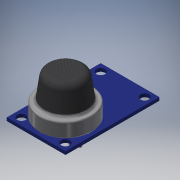
# Autodesk Inventor part: MQ_New
Saved by Autodesk Inventor 2019 (Build 230136000, 136)
## iProperties
Created: 2019-06-20
Part Number: MQ_New
Material: Steel, Mild, Welded
Document SubType Name: Modeling
Designer: hecto
Density: 7.85 g/cm^3
Appearance: Rubber - Blue(2)
Author: hecto
Autodesk Inventor part; units mm, degrees
ref_plane "YZ Plane" through (0, 0, 0) normal (1, 0, 0) x (0, 1, 0)
ref_plane "XZ Plane" through (0, 0, 0) normal (0, 1, 0) x (-1, 0, 0)
ref_plane "XY Plane" through (0, 0, 0) normal (0, 0, 1) x (1, 0, 0)
sketch "Sketch1" plane through (0, 0, 0) normal (0, 1, 0) x (-1, 0, 0)
  line L0 (10, -16) -> (-10, -16)
  line L1 (-10, -16) -> (-10, 16)
  line L2 (-10, 16) -> (10, 16)
  line L3 (10, 16) -> (10, -16)
  point P0 (0, 0)
  point P1 (0, -16)
  point P2 (10, 0)
  dimension "d0" = 20
  dimension "d1" = 32
  constraints: 8 end point, 2 midpoint, 2 parallel, 1 horizontal, 1 horizontal alignment, 1 perpendicular, 1 vertical alignment
  measures "d0" distance of L1.end L2.end
  measures "d1" distance of L0.end L1.end
extrude "Extrusion1" add sketch "Sketch1" along normal blind 1.1
sketch "Sketch2" plane through (0, 1.1, 0) normal (0, 1, 0) x (1, 0, 0)
  circle A0 centre (-7.5, -13.5) radius 1.5
  line L0 (-10, -16) -> (10, -16) projected
  line L1 (-10, 16) -> (-10, -16) projected
  line L2 (-10, 0) -> (10, 0) construction
  line L3 (0, -16) -> (0, 16)
  circle A1 centre (-7.5, 13.5) radius 1.5
  circle A2 centre (7.5, -13.5) radius 1.5
  circle A3 centre (7.5, 13.5) radius 1.5
  point P0 (0, 0)
  dimension "d4" = 3
  dimension "d5" = 2.5
  dimension "d6" = 2.5
  constraints: 4 centre point, 4 end point, 3 symmetric about line, 2 midpoint, 1 horizontal, 1 vertical, 3 other
  measures "d4" diameter of A0
  measures "d5" distance from line of L0 A0.centre
  measures "d6" distance from line of L1 A0.centre
extrude "Extrusion2" cut sketch "Sketch2" against normal through all
sketch "Sketch3" plane through (0, 1.1, 0) normal (0, 1, 0) x (1, 0, 0)
  circle A0 centre (0, -6) radius 9
  line L0 (-10, -16) -> (10, -16) projected
  point P0 (0, 0)
  dimension "d9" = 18
  dimension "d10" = 10
  constraints: 1 centre point, 1 vertical alignment
  measures "d9" diameter of A0
  measures "d10" distance from line of L0 A0.centre
extrude "Extrusion3" add sketch "Sketch3" along normal blind 5
fillet "Fillet1" radius 0.5 1 edges at (-9, 6.1, 6)
sketch "Sketch4" plane through (0, 0, 0) normal (1, 0, 0) x (0, 1, 0)
  line L0 (1.1, 15) -> (5.6, 15) construction
  line L1 (1.1, 15) -> (1.1, 12) construction
  arc A0 (6.1, 14.5) -> (5.6, 15) centre (5.6, 14.5) ccw projected
  line L2 (1.1, 15) -> (1.1, 12.0001) projected
  line L3 (1.1, 15) -> (1.6, 15)
  line L4 (1.1, 15) -> (1.1, 14.5)
  arc A1 (1.6, 15) -> (1.1, 14.5) centre (1.6, 14.5) ccw
  line L5 (6.1, 6) -> (3.5731, 6) construction
  line L6 (6.1, 14.5) -> (6.1, -2.5) construction
  point P0 (0, 0)
  point P1 (1.1, 6)
  dimension "d17" = 0.5
  dimension "d18" = 0.5
  constraints: 6 end point, 2 point on circle, 2 point on line, 1 centre point, 1 horizontal, 1 midpoint, 1 tangent
  measures "d17" distance of L0.start L3.end
  measures "d18" distance of L0.start L4.end
revolve "Revolution1" cut sketch "Sketch4" angle 360 about axis through (0, 6.1, 6) along (0, -1, 0)
sketch "Sketch5" plane through (0, 0, 0) normal (1, 0, 0) x (0, 1, 0)
  line L0 (13.274, 6) -> (6.1, 6)
  line L1 (6.1, 14.5) -> (6.1, -2.5) projected
  arc A0 (6.1, 14.166) -> (6.9626, 13.1755) centre (7.1, 14.166) ccw
  line L2 (13.274, 12.3) -> (13.274, 6)
  line L3 (13.274, 12.3) -> (6.9626, 13.1755)
  line L4 (6.1, 14.166) -> (6.1, 6)
  line L5 (14.9992, 10.319) -> (14.9992, 6)
  line L6 (13.274, 6) -> (14.9992, 6)
  arc A1 (14.9992, 10.319) -> (13.274, 12.3) centre (12.9992, 10.319) ccw
  point P0 (0, 0)
  point P1 (13.274, 10.9657)
  dimension "d20" = 2
  dimension "d21" = 0.334
  dimension "d22" = 7.174
  dimension "d23" = 6.3
  dimension "d35" = 4
  constraints: 12 end point, 4 point on circle, 4 tangent, 3 point on line, 2 centre point, 2 horizontal, 2 horizontal alignment, 2 midpoint, 2 vertical
  measures "d20" diameter of A0
  measures "d21" vertical distance of L1.start A0.centre
  measures "d22" distance of L0.start L0.end
  measures "d23" distance of L2.start L0.start
  measures "d35" diameter of A1
revolve "Revolution2" add sketch "Sketch5" angle 360 about axis through (0, 13.274, 6) along (0, -1, 0)
sketch "Sketch6" plane through (0, 0, 0) normal (0, -1, 0) x (1, 0, 0)
  circle A0 centre (0, 6) radius 7.166 projected
  circle A1 centre (0, 6) radius 5 construction
  circle A2 centre (5, 6) radius 0.5
  circle A3 centre (4.3301, 8.5) radius 0.5
  circle A4 centre (2.5, 10.3301) radius 0.5
  circle A5 centre (0, 11) radius 0.5
  circle A6 centre (-2.5, 10.3301) radius 0.5
  circle A7 centre (-4.3301, 8.5) radius 0.5
  circle A8 centre (-5, 6) radius 0.5
  circle A9 centre (-4.3301, 3.5) radius 0.5
  circle A10 centre (-2.5, 1.6699) radius 0.5
  circle A11 centre (0, 1) radius 0.5
  circle A12 centre (2.5, 1.6699) radius 0.5
  circle A13 centre (4.3301, 3.5) radius 0.5
  point P0 (0, 0)
  dimension "d27" = 10
  dimension "d28" = 1
  dimension "d31" = 360
  constraints: 12 centre point, 2 horizontal alignment, 1 coincident, 27 other
  measures "d28" diameter of A2
extrude "Extrusion4" add sketch "Sketch6" along normal blind 5 contours A2 | A3 | A7 | A8 | A9 | A13
sketch "Sketch7" plane through (0, 0, 0) normal (0, -1, 0) x (1, 0, 0)
  line L0 (5, -11) -> (-5, -11)
  line L1 (-5, -11) -> (-5, -13.5)
  line L2 (-5, -13.5) -> (5, -13.5)
  line L3 (5, -13.5) -> (5, -11)
  line L4 (-10, -16) -> (10, -16) projected
  point P0 (0, 0)
  point P1 (0, -13.5)
  dimension "d36" = 10
  dimension "d37" = 2.5
  dimension "d38" = 2.5
  constraints: 8 end point, 2 parallel, 1 horizontal, 1 midpoint, 1 perpendicular, 1 vertical alignment
  measures "d36" distance of L1.end L2.end
  measures "d37" distance of L2.end L0.start
  measures "d38" distance between parallel lines of L4 L2
extrude "Extrusion5" add sketch "Sketch7" along normal blind 2.5
sketch "Sketch8" plane through (0, -2.5, 0) normal (0, -1, 0) x (1, 0, 0)
  line L0 (4.2, -12.7) -> (3.3, -12.7)
  line L1 (3.3, -12.7) -> (3.3, -11.8)
  line L2 (3.3, -11.8) -> (4.2, -11.8)
  line L3 (4.2, -11.8) -> (4.2, -12.7)
  line L4 (5, -13.5) -> (5, -11) projected
  line L5 (5, -11) -> (-5, -11) projected
  line L6 (-5, -11) -> (-5, -13.5) projected
  line L7 (-5, -13.5) -> (5, -13.5) projected
  line L8 (5, -13.5) -> (5, -11) projected
  line L9 (1.7, -12.7) -> (0.8, -12.7)
  line L10 (1.7, -11.8) -> (1.7, -12.7)
  line L11 (0.8, -12.7) -> (0.8, -11.8)
  line L12 (0.8, -11.8) -> (1.7, -11.8)
  line L13 (-0.8, -12.7) -> (-1.7, -12.7)
  line L14 (-0.8, -11.8) -> (-0.8, -12.7)
  line L15 (-1.7, -12.7) -> (-1.7, -11.8)
  line L16 (-1.7, -11.8) -> (-0.8, -11.8)
  line L17 (-3.3, -12.7) -> (-4.2, -12.7)
  line L18 (-3.3, -11.8) -> (-3.3, -12.7)
  line L19 (-4.2, -12.7) -> (-4.2, -11.8)
  line L20 (-4.2, -11.8) -> (-3.3, -11.8)
  point P0 (0, 0)
  point P1 (5, -12.25)
  point P2 (4.2, -12.25)
  point P3 (1.7, -12.25)
  point P4 (-0.8, -12.25)
  point P5 (-3.3, -12.25)
  dimension "d41" = 0.9
  dimension "d42" = 0.9
  dimension "d43" = 0.8
  dimension "d46" = 2.5
  constraints: 32 end point, 2 horizontal, 2 midpoint, 2 parallel, 1 horizontal alignment, 1 perpendicular, 27 other
  measures "d41" distance of L1.end L2.end
  measures "d42" distance of L0.end L1.end
  measures "d43" distance between parallel lines of L4 L3
  measures "d46" distance of L0.start L9.start
extrude "Extrusion6" add sketch "Sketch8" along normal blind 2 contours L0 L1 L2 L3 | L9 L11 L12 L10 | L13 L15 L16 L14 | L17 L19 L20 L18
sketch "Sketch9" plane through (4.2, -2.5, -12.7) normal (0, 0, -1) x (-1, 0, 0)
  line L0 (0, 0) -> (0.9, 0) projected
  line L1 (0, 0) -> (0, -2) projected
  line L2 (0.9, -2) -> (0, -2) projected
  line L3 (0.9, 0) -> (0.9, -2) projected
  line L4 (0.9, -1.1) -> (0, -1.1)
  point P0 (4.2, 2.5)
  dimension "d53" = 0.9
  dimension "d54" = 0.9
  constraints: 2 end point, 2 point on line, 1 horizontal
  measures "d53" distance between parallel lines of L4 L2
  measures "d54" distance of L2.start L1.end
extrude "Extrusion7" add sketch "Sketch9" along normal blind 8 contours L4 L3 L2 L1
chamfer "Chamfer1" distance 0.3 angle 45 4 edges at (4.2, -4.05, -20.7) (3.75, -4.5, -20.7) (3.3, -4.05, -20.7) (3.75, -3.6, -20.7)
pattern_linear "Rectangular Pattern1" count 4 spacing 2.5 along (-1, 0, 0) of "Extrusion7", "Chamfer1"
equation "\"d53\" = d54"
body "Solid1"
